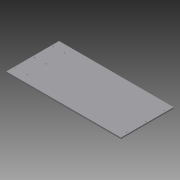
# Autodesk Inventor part: large wall
Saved by Autodesk Inventor 2015 (Build 190159000, 159)
## iProperties
Created: 2015-01-31
Part Number: large wall
Material: Generic
Document SubType Name: Modeling
Designer: Joseph
Density: 1 g/cm^3
Appearance: Default
Author: Joseph
Autodesk Inventor part; units mm, degrees
ref_plane "YZ Plane" through (0, 0, 0) normal (1, 0, 0) x (0, 1, 0)
ref_plane "XZ Plane" through (0, 0, 0) normal (0, 1, 0) x (-1, 0, 0)
ref_plane "XY Plane" through (0, 0, 0) normal (0, 0, 1) x (1, 0, 0)
sketch "Sketch1" plane through (0, 0, 0) normal (0, 0, 1) x (1, 0, 0)
  line L0 (0, -18.0326) -> (20, -18.0326) projected
  line L1 (20, 0) -> (20, -18.0326) projected
  line L2 (-580, 258.0326) -> (-500, 258.0326) projected
  line L3 (-580, 240) -> (-580, 258.0326) projected
  line L4 (20, -18.0326) -> (-580, -18.0326)
  line L5 (-580, -18.0326) -> (-580, 258.0326)
  line L6 (-580, 258.0326) -> (20, 258.0326)
  line L7 (20, 258.0326) -> (20, -18.0326)
  point P0 (0, 0)
  constraints: 8 end point, 2 parallel, 1 horizontal, 1 perpendicular
extrude "Extrusion1" add sketch "Sketch1" along normal blind 6.35
sketch "Sketch2" plane through (0, 0, 6.35) normal (0, 0, 1) x (1, 0, 0)
  line L0 (-580, -18.0326) -> (20, -18.0326) projected
  line L1 (20, -18.0326) -> (20, 258.0326) projected
  line L2 (20, 258.0326) -> (-580, 258.0326) projected
  line L3 (-580, 258.0326) -> (-580, -18.0326) projected
  circle A0 centre (20, 120) radius 10 construction
  line L4 (10, 258.0326) -> (10, -18.0326) construction
  circle A1 centre (10, 258.0326) radius 40 construction
  circle A2 centre (10, -18.0326) radius 40 construction
  line L5 (10, 218.0326) -> (-580, 218.0326) construction
  line L6 (10, 120) -> (-580, 120) construction
  line L7 (10, 21.9674) -> (-580, 21.9674) construction
  circle A3 centre (-580, 120) radius 10 construction
  circle A4 centre (-580, 120) radius 70 construction
  line L8 (-570, 258.0326) -> (-570, -18.0326) construction
  line L9 (-510, 258.0326) -> (-510, -18.0326) construction
  point P0 (0, 0)
  point P1 (-510, 218.0326)
  point P2 (-570, 218.0326)
  point P3 (-570, 120)
  point P4 (-510, 120)
  point P5 (-510, 21.9674)
  point P6 (-570, 21.9674)
  dimension "d3" = 80
  dimension "d4" = 80
  dimension "d2" = 20
  dimension "d5" = 20
  dimension "d6" = 140
  constraints: 18 point on line, 12 end point, 5 midpoint, 4 coincident, 3 centre point, 3 perpendicular, 2 horizontal, 2 vertical alignment, 1 parallel, 1 vertical, 4 other
  measures "d2" diameter of A0
  measures "d5" diameter of A3
  measures "d6" diameter of A4
hole "Hole1" at (10, 120, 6.35) at (10, 218.0326, 6.35) at (10, 21.9674, 6.35) at (-510, 218.0326, 6.35) at (-570, 218.0326, 6.35) at (-570, 120, 6.35) at (-510, 120, 6.35) at (-510, 21.9674, 6.35) at (-570, 21.9674, 6.35) direction (0, 0, -1) diameter 4.5 end through all clearance for "Socket Head Cap Screw" size "M4" standard "Ansi Metric M Profile"
body "Solid1"
